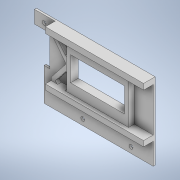
# Autodesk Inventor part: gen2-hdmi-mount
Saved by Autodesk Inventor 2021 (Build 250183000, 183)
## iProperties
Created: 2026-03-24
Part Number: gen2-hdmi-mount
Material: Generic
Document SubType Name: Sheet Metal
Designer: Toby
Density: 1 g/cm^3
Sheet Metal Rule: Default_mm
Appearance: Default
Author: Toby
Autodesk Inventor part; units mm, degrees
ref_plane "YZ Plane" through (0, 0, 0) normal (1, 0, 0) x (0, 1, 0)
ref_plane "XZ Plane" through (0, 0, 0) normal (0, 1, 0) x (-1, 0, 0)
ref_plane "XY Plane" through (0, 0, 0) normal (0, 0, 1) x (1, 0, 0)
sketch "Sketch1" plane through (0, 0, 0) normal (0, 0, 1) x (1, 0, 0)
  line L0 (-40.83, 19.81) -> (40.83, 19.81)
  line L1 (40.83, 19.81) -> (40.83, -19.81)
  line L2 (40.83, -19.81) -> (-40.83, -19.81)
  line L3 (-40.83, -19.81) -> (-40.83, 19.81)
  point P0 (0, 0)
  dimension "d0" = 81.66
  dimension "d1" = 39.62
  dimension "d2" = 19.81
  dimension "d3" = 40.83
  constraints: 8 end point, 2 parallel, 1 horizontal, 1 perpendicular
  measures "d0" distance of L0.start L0.end
  measures "d1" distance of L2.end L0.start
  measures "d2" distance from line of point (0, 0) L0
  measures "d3" distance from line of point (0, 0) L3
extrude "Extrusion1" add sketch "Sketch1" along normal blind 1
sketch "Sketch2" plane through (0, 0, 1) normal (0, 0, 1) x (1, 0, 0)
  line L0 (-40.83, 19.81) -> (-40.83, -19.81) projected
  line L1 (-40.83, -19.81) -> (40.83, -19.81) projected
  point P0 (0, 0)
  point P1 (-15.83, 16.19)
  point P2 (4.17, -16.81)
  point P3 (29.17, -16.81)
  dimension "d6" = 25
  dimension "d7" = 36
  dimension "d8" = 45
  dimension "d9" = 3
  dimension "d10" = 3
  dimension "d11" = 70
  measures "d6" distance from line of L0 point (-15.83, 16.19)
  measures "d7" distance from line of L1 point (-15.83, 16.19)
  measures "d8" distance from line of L0 point (4.17, -16.81)
  measures "d9" distance from line of L1 point (4.17, -16.81)
  measures "d10" distance from line of L1 point (29.17, -16.81)
  measures "d11" distance from line of L0 point (29.17, -16.81)
hole "Hole1" at (-15.83, 16.19, 1) at (4.17, -16.81, 1) at (29.17, -16.81, 1) direction (0, 0, -1) diameter 2 depth 3 tip angle 118
sketch "Sketch3" plane through (0, 0, 1) normal (0, 0, 1) x (1, 0, 0)
  line L0 (-40.83, 19.81) -> (-40.83, -19.81) projected
  line L1 (-40.83, 13.19) -> (-12.83, 13.19)
  line L2 (-12.83, 13.19) -> (-12.83, -2.81)
  line L3 (-12.83, -2.81) -> (-40.83, -2.81)
  line L4 (-40.83, -2.81) -> (-40.83, 13.19)
  line L5 (-40.83, -19.81) -> (40.83, -19.81) projected
  line L6 (40.83, 19.81) -> (-40.83, 19.81) projected
  line L7 (-40.83, 19.81) -> (-20.83, 19.81)
  line L8 (-20.83, 19.81) -> (-20.83, 13.19)
  line L9 (-20.83, 13.19) -> (-40.83, 13.19)
  line L10 (-40.83, 13.19) -> (-40.83, 19.81)
  line L11 (-40.83, -19.81) -> (40.83, -19.81) projected
  line L12 (40.83, -19.81) -> (40.83, 19.81) projected
  line L13 (-20.83, 19.81) -> (40.83, 19.81)
  line L14 (40.83, 19.81) -> (40.83, -19.81)
  line L15 (40.83, -19.81) -> (-20.83, -19.81)
  line L16 (-20.83, -19.81) -> (-20.83, 19.81)
  line L17 (-40.83, -2.81) -> (-20.83, -2.81)
  line L18 (-20.83, -2.81) -> (-20.83, -19.81)
  line L19 (-20.83, -19.81) -> (-40.83, -19.81)
  line L20 (-40.83, -19.81) -> (-40.83, -2.81)
  point P0 (0, 0)
  point P1 (-0.83, -19.81)
  point P2 (-20.83, -2.81)
  dimension "d19" = 28
  dimension "d20" = 33
  dimension "d21" = 17
  dimension "d22" = 8
  constraints: 32 end point, 8 parallel, 4 horizontal, 4 perpendicular, 2 point on line
  measures "d19" distance of L1.start L1.end
  measures "d20" distance between parallel lines of L5 L1
  measures "d21" distance between parallel lines of L5 L3
  measures "d22" distance between parallel lines of L2 L8
extrude "Extrusion2" cut sketch "Sketch3" against normal blind 1 contours L6 L8 L1 L0 | L1 L16 L3 L0 | L3 L16 L5 L0 | L1 L2 L3 L16
sketch "Sketch4" plane through (0, 0, 1) normal (0, 0, 1) x (1, 0, 0)
  line L0 (-12.83, -2.81) -> (-20.83, -2.81) projected
  line L1 (-20.83, -2.81) -> (-20.83, -19.81) projected
  line L2 (-15.83, -2.81) -> (-20.83, -2.81)
  line L3 (-20.83, -2.81) -> (-20.83, -19.81)
  line L4 (-20.83, -19.81) -> (-15.83, -19.81)
  line L5 (-15.83, -19.81) -> (-15.83, -2.81)
  line L6 (-12.83, 13.19) -> (-12.83, -2.81) projected
  point P0 (0, 0)
  dimension "d26" = 3
  constraints: 8 end point, 2 parallel, 1 horizontal, 1 perpendicular, 1 point on line
  measures "d26" distance between parallel lines of L5 L6
extrude "Extrusion3" cut sketch "Sketch4" against normal blind 1
sketch "Sketch5" plane through (0, 0, 1) normal (0, 0, 1) x (1, 0, 0)
  line L0 (-1.17, 16.81) -> (30.83, 16.81)
  line L1 (30.83, 16.81) -> (30.83, -5.81)
  line L2 (30.83, -5.81) -> (-1.17, -5.81)
  line L3 (-1.17, -5.81) -> (-1.17, 16.81)
  line L4 (40.83, -19.81) -> (40.83, 19.81) projected
  line L5 (40.83, 19.81) -> (-20.83, 19.81) projected
  line L6 (-15.83, -19.81) -> (40.83, -19.81) projected
  point P0 (0, 0)
  dimension "d29" = 10
  dimension "d30" = 42
  dimension "d31" = 3
  dimension "d32" = 14
  constraints: 8 end point, 2 parallel, 1 horizontal, 1 perpendicular
  measures "d29" distance between parallel lines of L4 L1
  measures "d30" distance between parallel lines of L4 L3
  measures "d31" distance between parallel lines of L0 L5
  measures "d32" distance between parallel lines of L6 L2
extrude "Extrusion4" add sketch "Sketch5" along normal blind 3
sketch "Sketch6" plane through (0, 0, 4) normal (0, 0, 1) x (1, 0, 0)
  line L0 (0.83, 11.81) -> (28.83, 11.81)
  line L1 (28.83, 11.81) -> (28.83, -0.81)
  line L2 (28.83, -0.81) -> (0.83, -0.81)
  line L3 (0.83, -0.81) -> (0.83, 11.81)
  line L4 (-1.17, 16.81) -> (-1.17, -5.81) projected
  line L5 (30.83, -5.81) -> (30.83, 16.81) projected
  line L6 (30.83, 16.81) -> (-1.17, 16.81) projected
  line L7 (-1.17, -5.81) -> (30.83, -5.81) projected
  point P0 (0, 0)
  dimension "d35" = 2
  dimension "d36" = 2
  dimension "d37" = 5
  dimension "d38" = 5
  constraints: 8 end point, 2 parallel, 1 horizontal, 1 perpendicular
  measures "d35" distance between parallel lines of L4 L3
  measures "d36" distance between parallel lines of L5 L1
  measures "d37" distance between parallel lines of L6 L0
  measures "d38" distance between parallel lines of L7 L2
extrude "Extrusion5" cut sketch "Sketch6" against normal blind 4 contours L0 L1 L2 L3
sketch "Sketch7" plane through (0, 0, 1) normal (0, 0, 1) x (1, 0, 0)
  line L0 (40.83, -19.81) -> (40.83, 19.81) projected
  line L1 (-10.17, -5.81) -> (40.83, -5.81)
  line L2 (40.83, -5.81) -> (40.83, -8.61)
  line L3 (40.83, -8.61) -> (-10.17, -8.61)
  line L4 (-10.17, -8.61) -> (-10.17, -5.81)
  line L5 (40.83, 19.81) -> (-20.83, 19.81) projected
  line L6 (-10.17, 19.81) -> (40.83, 19.81)
  line L7 (40.83, 19.81) -> (40.83, 16.81)
  line L8 (40.83, 16.81) -> (-10.17, 16.81)
  line L9 (-10.17, 16.81) -> (-10.17, 19.81)
  line L10 (30.83, 16.81) -> (-1.17, 16.81) projected
  line L11 (-1.17, -5.81) -> (30.83, -5.81) projected
  point P0 (0, 0)
  point P1 (40.83, -5.81)
  dimension "d41" = 3
  dimension "d42" = 51
  dimension "d43" = 2.8
  constraints: 16 end point, 4 parallel, 3 collinear, 3 point on line, 2 horizontal, 2 perpendicular
  measures "d41" distance between parallel lines of L5 L8
  measures "d42" distance between parallel lines of L0 L9
  measures "d43" distance between parallel lines of L1 L3
extrude "Extrusion6" add sketch "Sketch7" along normal blind 5
sketch "Sketch8" plane through (40.83, -19.81, 0) normal (1, 0, 0) x (0, 0, -1)
  line L0 (0, 0) -> (0, 39.62) projected
  line L1 (0, 0) -> (-6, 0)
  line L2 (-6, 0) -> (-6, 39.62)
  line L3 (-6, 39.62) -> (0, 39.62)
  line L4 (0, 39.62) -> (0, 0)
  point P0 (0, 19.81)
  constraints: 8 end point, 2 parallel, 1 horizontal, 1 perpendicular
extrude "Extrusion7" cut sketch "Sketch8" against normal blind 0.2
sketch "Sketch9" plane through (0, 0, 1) normal (0, 0, 1) x (1, 0, 0)
  line L0 (-10.17, 16.81) -> (40.63, 16.81) projected
  line L1 (-10.17, 16.81) -> (-1.17, 5.5) construction
  line L2 (-1.17, 16.81) -> (-1.17, -5.81) projected
  line L3 (-10.9525, 16.1873) -> (-1.9525, 4.8773)
  line L4 (-0.3875, 6.1227) -> (-9.3875, 17.4327)
  arc A0 (-9.3875, 17.4327) -> (-10.9525, 16.1873) centre (-10.17, 16.81) ccw
  arc A1 (-1.9525, 4.8773) -> (-0.3875, 6.1227) centre (-1.17, 5.5) ccw
  line L5 (-10.17, -5.81) -> (-1.17, -5.81) projected
  line L6 (-1.17, 5.5) -> (-10.17, -5.81) construction
  line L7 (-1.9525, 6.1227) -> (-10.9525, -5.1873)
  line L8 (-9.3875, -6.4327) -> (-0.3875, 4.8773)
  arc A2 (-0.3875, 4.8773) -> (-1.9525, 6.1227) centre (-1.17, 5.5) ccw
  arc A3 (-10.9525, -5.1873) -> (-9.3875, -6.4327) centre (-10.17, -5.81) ccw
  line L9 (-10.17, 19.81) -> (-10.17, 16.81) projected
  line L10 (-10.17, 19.81) -> (-10.17, -8.4856)
  point P0 (0, 0)
  point P1 (-5.67, 11.155)
  point P2 (-5.67, -0.155)
  point P3 (-10.17, 15.204)
  point P4 (-2.448, 5.5)
  point P5 (-10.17, -4.204)
  point P6 (-8.892, -5.81)
  point P7 (-1.17, 3.894)
  point P8 (-1.17, 7.106)
  point P9 (-8.892, 16.81)
  dimension "d48" = 2
  dimension "d49" = 2
  constraints: 18 end point, 8 point on circle, 8 tangent, 4 centre point, 3 midpoint, 2 parallel, 1 vertical
  measures "d48" diameter of A1
  measures "d49" diameter of A3
extrude "Extrusion8" add sketch "Sketch9" along normal blind 2 contours L0 L4 L2 A2 L7 L3 L10 | L7 A2 L2 A1 L3 | L3 A1 L2 L8 L5 L10 L7
fillet "Fillet1" radius 1 6 edges at (-8.892, 16.81, 2) (-1.17, 7.106, 2) (-1.17, 16.81, 2.5) (-1.17, 3.894, 2) (-8.892, -5.81, 2) (-1.17, -5.81, 2.5)
fillet "Fillet2" radius 1 1 edges at (-2.448, 5.5, 2)
equation "\"BendRadius\" = Thickness"
equation "\"BendReliefWidth\" = Thickness"
equation "\"BendReliefDepth\" = 0.5 * Thickness"
equation "\"CornerReliefSize\" = 4 * Thickness"
equation "\"MinimumRemnant\" = 2 * Thickness"
equation "\"TransitionRadius\" = BendRadius"
equation "\"JacobiRadiusSize\" = BendRadius"
equation "\"GapSize\" = Thickness"
equation "\"Thickness\" = 0.5"
body "Solid1"
